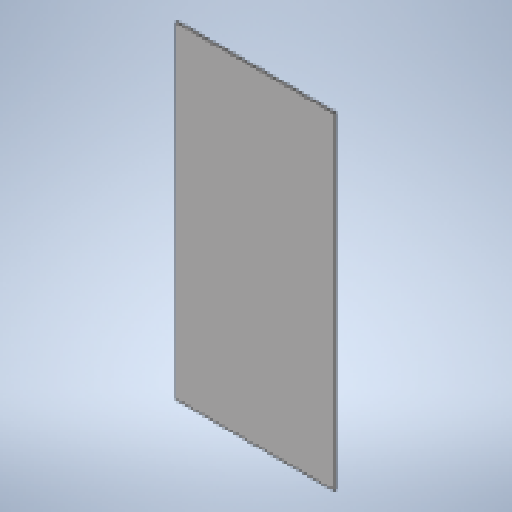
# Autodesk Inventor part: MSC 709 ridge 5
Saved by Autodesk Inventor 2025 (Build 290162010, 162A)
## iProperties
Created: 2024-06-20
Part Number: MSC 709 ridge 5
Material: Stainless Steel
Document SubType Name: Sheet Metal
Designer: pokla
Stock Number: МОО 709 пила 5
Density: 8 g/cm^3
Sheet Metal Rule: AISI304 2mm Die12
Appearance: Default
Flat Pattern Width: 19.4 cm
Flat Pattern Length: 40 cm
Flat Pattern Area: 776 cm^2
Sheet Metal Width: 194,000 mm
Sheet Metal Length: 400,000 mm
Sheet Metal Area: 77600,000 mm^2
Author: pokla
Autodesk Inventor part; units mm, degrees
ref_plane "YZ Plane" through (0, 0, 0) normal (1, 0, 0) x (0, 1, 0)
ref_plane "XZ Plane" through (0, 0, 0) normal (0, 1, 0) x (-1, 0, 0)
ref_plane "XY Plane" through (0, 0, 0) normal (0, 0, 1) x (1, 0, 0)
sketch "Sketch1" plane through (0, 0, 0) normal (0, 1, 0) x (-1, 0, 0)
  line L0 (0, 200) -> (-194, 200)
  line L1 (-194, 200) -> (-194, -200)
  line L2 (-194, -200) -> (0, -200)
  line L3 (0, -200) -> (0, 200)
  point P0 (0, 0)
  point P1 (0, 0)
  dimension "d0" = 400
  dimension "d1" = 194
  measures "d0" distance of L2.end L0.start
  measures "d1" distance of L1.end L2.end
extrude "Plate2" add sketch "Sketch1" along normal blind 2
equation "\"d3\" = Thickness"
equation "\"BendReliefWidth\" = Thickness"
equation "\"BendReliefDepth\" = 0.5 * Thickness"
equation "\"CornerReliefSize\" = 4 * Thickness"
equation "\"MinimumRemnant\" = 2 * Thickness"
equation "\"TransitionRadius\" = BendRadius"
equation "\"JacobiRadiusSize\" = BendRadius"
equation "\"GapSize\" = Thickness"
equation "\"Thickness\" = 2"
equation "\"BendRadius\" = 2.5"
body "Solid2"
